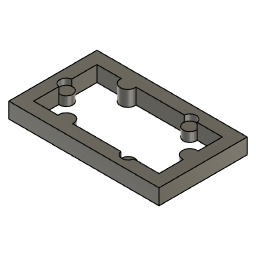
grove_2x1_sensor_mount (Autodesk Fusion 360 design; units mm, degrees)
Autodesk Fusion 360 part; units mm, degrees
sketch "Sketch1" plane through (0, 0, 0) normal (0, 0, 1) x (1, 0, 0)
  line L0 (24.2, -14.2) -> (-24.2, -14.2)
  line L1 (-24.2, -14.2) -> (-24.2, 14.2)
  line L2 (-24.2, 14.2) -> (24.2, 14.2)
  line L3 (24.2, 14.2) -> (24.2, -14.2)
  line L4 (24.2, -14.2) -> (-24.2, 14.2) construction
  line L5 (-24.2, -14.2) -> (24.2, 14.2) construction
  dimension "d1" = 48.4
  dimension "d2" = 28.4
  constraint horizontal L0
  constraint perpendicular L0 L1
  constraint parallel L0 L2
  constraint parallel L1 L3
  constraint coincident L4 origin
  constraint coincident L5 origin
  measures "d1" distance of L1.end L2.end
  measures "d2" distance of L0 L2
extrude "Extrude1" add sketch "Sketch1" along normal blind 5
shell "Shell1" thickness 4 removed faces 2 at (-8.0667, -4.7333, 5) at (-8.0667, -4.7333, 0)
sketch "Sketch2" plane through (0, 0, 5) normal (0, 0, 1) x (-1, 0, 0)
  line L0 (-20.2, -10.2) -> (-20.2, 10.2)
  line L1 (-20.2, 10.2) -> (20.2, 10.2)
  line L2 (20.2, 10.2) -> (20.2, -10.2)
  line L3 (20.2, -10.2) -> (-20.2, -10.2)
  line L4 (-24.2, -14.2) -> (24.2, -14.2)
  line L5 (24.2, -14.2) -> (24.2, 14.2)
  line L6 (24.2, 14.2) -> (-24.2, 14.2)
  line L7 (-24.2, 14.2) -> (-24.2, -14.2)
  circle A0 centre (19.9, 0) radius 2.1
  circle A1 centre (10, -9.9) radius 2.4
  circle A2 centre (-10, -9.9) radius 2.1
  circle A3 centre (-19.9, 0) radius 2.4
  line L8 (-20.2, 0) -> (20.2, 0) construction
  line L9 (0, -10.2) -> (0, 10.2) construction
  circle A4 centre (-10, 9.9) radius 2.1
  circle A5 centre (10, 9.9) radius 2.4
  dimension "d6" = 4.2
  dimension "d7" = 0.3
  dimension "d8" = 4.8
  dimension "d9" = 0.3
  dimension "d11" = 4.2
  dimension "d12" = 0.3
  dimension "d14" = 4.8
  dimension "d15" = 0.3
  dimension "d16" = 10
  dimension "d17" = 10
  dimension "d18" = 4.2
  dimension "d19" = 0.3
  dimension "d20" = 10
  dimension "d21" = 4.8
  dimension "d22" = 10
  dimension "d23" = 0.3
  constraint midpoint L0 L8.start
  constraint midpoint L2 L8.end
  constraint midpoint L3 L9.start
  constraint midpoint L1 L9.end
  measures "d6" diameter of A0
  measures "d7" distance of L2 A0.centre
  measures "d8" diameter of A1
  measures "d9" distance of L3 A1.centre
  measures "d11" diameter of A2
  measures "d12" distance of L3 A2.centre
  measures "d14" diameter of A3
  measures "d15" distance of L0 A3.centre
  measures "d16" distance of A2.centre L9
  measures "d17" distance of A1.centre L9
  measures "d18" diameter of A4
  measures "d19" distance of L1 A4.centre
  measures "d20" distance of L9 A4.centre
  measures "d21" diameter of A5
  measures "d22" distance of L9 A5.centre
  measures "d23" distance of L1 A5.centre
extrude "Extrude2" add sketch "Sketch2" against normal blind 5 contours L0 A3 | L3 A1 | L1 A5 picked at (-19.3318, 0.2231) picked at (10.663, -9.6523) picked at (10.9063, 9.3029)
extrude "Extrude3" cut sketch "Sketch2" against normal blind 2 contours L3 A2 | L1 A4 | L2 A0 picked at (-9.6779, -10.88) picked at (-10.1971, 10.7717) picked at (20.7929, -0.0996)
extrude "Extrude4" add sketch "Sketch2" against normal blind 3 from surface at -2 contours L3 A2 | L1 A4 | L2 A0 picked at (-9.4862, -9.6246) picked at (-9.7428, 9.449) picked at (19.4174, -0.1552)
